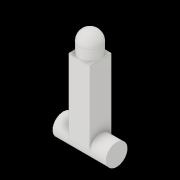
# Autodesk Inventor part: L3_0.1
Saved by Autodesk Inventor 2019 (Build 230136000, 136)
## iProperties
Created: 2021-08-06
Part Number: L3_0.1
Material: ABS 플라스틱
Document SubType Name: Modeling
Designer: YoonJunHeon
Density: 1.06 g/cm^3
Appearance: 매끄러움 - 흰색
Mass: 48550.5 g
Surface Area: 9769.91 cm^2
Volume: 45802.4 cm^3
Author: YoonJunHeon
Autodesk Inventor part; units mm, degrees
ref_plane "YZ Plane" through (0, 0, 0) normal (1, 0, 0) x (0, 1, 0)
ref_plane "XZ Plane" through (0, 0, 0) normal (0, 1, 0) x (-1, 0, 0)
ref_plane "XY Plane" through (0, 0, 0) normal (0, 0, 1) x (1, 0, 0)
sketch "스케치5" plane through (0, 0, 0) normal (1, 0, 0) x (0, 1, 0)
  circle A0 centre (0, 0) radius 10
  dimension "d11" = 20
  constraints: 1 centre point, 1 coincident
  measures "d11" diameter of A0
extrude "돌출4" add sketch "스케치5" along normal mid plane 50
sketch "스케치6" plane through (0, 0, 0) normal (0, 1, 0) x (-1, 0, 0)
  line L0 (25, 10) -> (-25, 10) projected
  line L1 (25, -10) -> (-25, -10) projected
  line L2 (-10, 10) -> (10, 10)
  line L3 (10, 10) -> (10, -10)
  line L4 (10, -10) -> (-10, -10)
  line L5 (-10, -10) -> (-10, 10)
  line L6 (25, -10) -> (25, 10) projected
  point P0 (0, 0)
  dimension "d14" = 20
  dimension "d15" = 15
  constraints: 8 end point, 2 parallel, 2 point on line, 1 horizontal, 1 perpendicular
  measures "d14" distance of L3.end L4.end
  measures "d15" distance between parallel lines of L3 L6
extrude "돌출5" add sketch "스케치6" along normal blind 70 contours L3 L1 L5 L0
sketch "스케치7" plane through (0, 70, 0) normal (0, 1, 0) x (1, 0, 0)
  circle A0 centre (0, 0) radius 10
  dimension "d18" = 20
  constraints: 1 centre point, 1 coincident
  measures "d18" diameter of A0
extrude "돌출6" add sketch "스케치7" along normal blind 10
sketch "스케치8" plane through (0, 80, 0) normal (0, 1, 0) x (1, 0, 0)
  circle A0 centre (0, 0) radius 10 projected
  line L0 (10, -10) -> (10, 0) projected
  line L1 (-10, 0) -> (10, 0)
  constraints: 2 end point, 1 horizontal, 1 point on circle
revolve "회전2" add sketch "스케치8" angle 360 about axis through (-10, 80, 0) along (1, 0, 0) picked at (2.495, 2.2104) contours L1 A0
